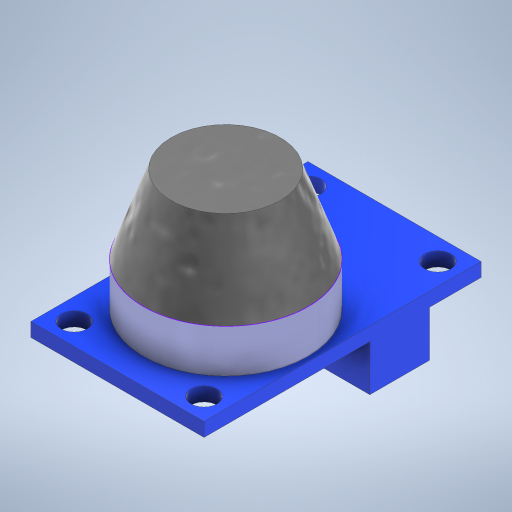
# Autodesk Inventor part: SensorGas
Saved by Autodesk Inventor 2024 (Build 280153000, 153)
## iProperties
Created: 2024-05-07
Part Number: SensorGas
Material: Genérico
Document SubType Name: Modeling
Designer: alexa
Density: 1 g/cm^3
Appearance: Valor por defecto
Author: alexa
Autodesk Inventor part; units mm, degrees
ref_plane "YZ Plane" through (0, 0, 0) normal (1, 0, 0) x (0, 1, 0)
ref_plane "XZ Plane" through (0, 0, 0) normal (0, 1, 0) x (-1, 0, 0)
sketch "Sketch1" plane through (0, 0, 0) normal (0, 1, 0) x (-1, 0, 0)
  line L0 (-10, 16) -> (10, 16)
  line L1 (10, 16) -> (10, -16)
  line L2 (10, -16) -> (-10, -16)
  line L3 (-10, -16) -> (-10, 16)
  line L4 (-10, 16) -> (10, -16) construction
  line L5 (10, 16) -> (-10, -16) construction
  point P0 (0, 0)
  dimension "d0" = 20
  dimension "d1" = 32
  constraints: 12 end point, 2 midpoint, 2 parallel, 1 horizontal, 1 perpendicular
  measures "d0" distance of L1.end L2.end
  measures "d1" distance of L0.end L1.end
extrude "Extrusion1" add sketch "Sketch1" along normal blind 1.6
sketch "Sketch3" plane through (0, 1.6, 0) normal (0, 1, 0) x (1, 0, 0)
  line L0 (-10, 16) -> (-10, -16) projected
  line L1 (-10, -16) -> (-7.5, -16)
  line L2 (-10, -16) -> (10, -16) projected
  line L3 (-7.5, -16) -> (-7.5, -13.5)
  circle A0 centre (-7.5, -13.5) radius 1.5
  point P0 (0, 0)
  dimension "d4" = 2.5
  dimension "d5" = 2.5
  dimension "d6" = 3
  constraints: 4 end point, 1 centre point, 1 coincident, 1 point on line, 1 vertical
  measures "d4" distance of L0.end L1.end
  measures "d5" distance of L1.end L3.end
  measures "d6" diameter of A0
extrude "Extrusion2" cut sketch "Sketch3" against normal blind 1.6
pattern_linear "Rectangular Pattern1" count 2 spacing 27 along (0, 0, -1) count 2 spacing 15 along (1, 0, 0) of "Extrusion2"
sketch "Sketch4" plane through (0, 1.6, 0) normal (0, 1, 0) x (1, 0, 0)
  line L0 (-10, -16) -> (10, -16) projected
  line L1 (10, 16) -> (-10, 16) projected
  circle A0 centre (0, -3.5) radius 9.5
  point P0 (0, 0)
  constraints: 1 centre point
extrude "Extrusion3" add sketch "Sketch4" along normal blind 5
ref_plane "Work Plane1" through (0, 15.6, 3.5) normal (0, 1, 0) x (1, 0, 0)
sketch "Sketch5" plane through (0, 15.6, 3.5) normal (0, 1, 0) x (1, 0, 0)
  circle A0 centre (0, 0) radius 6.3
  point P0 (0, 3.5)
  dimension "d22" = 12.6
  constraints: 1 centre point
  measures "d22" diameter of A0
sketch "Sketch6" plane through (0, 6.6, 3.5) normal (0, 1, 0) x (1, 0, 0)
  circle A0 centre (0, 0) radius 9.5
  point P0 (0, 3.5)
  constraints: 1 centre point
loft "Loft1" add profiles "Sketch5" section 1 edges at (-9.5, 6.6, 3.5)
sketch "Sketch7" plane through (0, 0, 0) normal (0, -1, 0) x (1, 0, 0)
  line L0 (9.9296, -16.0477) -> (10, -10.0481)
  line L1 (10, 16) -> (10, -16) projected
  line L2 (10, -10.0481) -> (3, -10.0481)
  line L3 (3, -10.0481) -> (3, -3.1481)
  line L4 (3, -3.1481) -> (10, -3.1481)
  line L5 (10, -3.1481) -> (10, -10.0481)
  point P0 (0, 0)
  dimension "d27" = 6
  dimension "d28" = 7
  dimension "d29" = 6.9
  constraints: 10 end point, 2 parallel, 1 horizontal, 1 perpendicular, 1 point on line
  measures "d27" distance of L0.start L0.end
  measures "d28" distance of L3.end L4.end
  measures "d29" distance of L2.end L3.end
extrude "Extrusion4" add sketch "Sketch7" along normal blind 5.3
body "Solid1"
